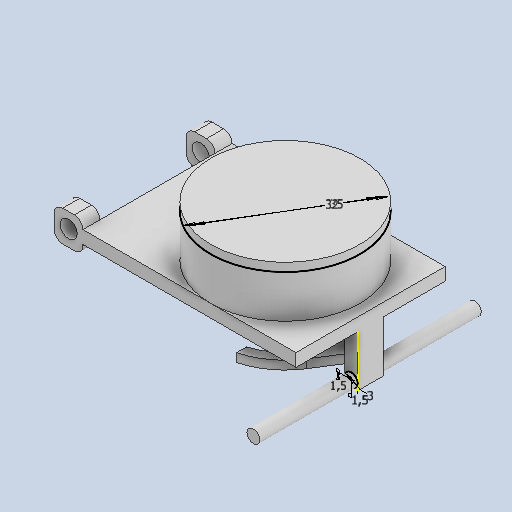
# Autodesk Inventor part: lid
Saved by Autodesk Inventor 2025 (Build 290162000, 162)
## iProperties
Created: 2025-08-06
Part Number: lid
Material: Generic
Document SubType Name: Modeling
Designer: Pravoslav
Density: 1 g/cm^3
Appearance: Default
Author: Pravoslav
Autodesk Inventor part; units mm, degrees
ref_plane "YZ Plane" through (0, 0, 0) normal (1, 0, 0) x (0, 1, 0)
ref_plane "XZ Plane" through (0, 0, 0) normal (0, 1, 0) x (-1, 0, 0)
ref_plane "XY Plane" through (0, 0, 0) normal (0, 0, 1) x (1, 0, 0)
sketch "Sketch1" plane through (0, 0, 0) normal (0, 1, 0) x (-1, 0, 0)
  circle A0 centre (0, 0) radius 16
  circle A1 centre (0, 0) radius 17.5
  dimension "d0" = 32
  dimension "d1" = 35
  constraints: 2 centre point, 2 coincident
  measures "d0" diameter of A0
  measures "d1" diameter of A1
extrude "Extrusion1" add sketch "Sketch1" along normal blind 2 contours A0 | A1
extrude "Extrusion2" add sketch "Sketch1" against normal blind 13
sketch "Sketch2" plane through (0, -13, 0) normal (0, -1, 0) x (1, 0, 0)
  line L0 (20, -17.5) -> (-30, -17.5)
  line L1 (-30, -17.5) -> (-30, 17.5)
  line L2 (-30, 17.5) -> (20, 17.5)
  line L3 (20, 17.5) -> (20, -17.5)
  circle A0 centre (0, 0) radius 17.5 projected
  point P0 (20, 0)
  point P1 (0, 17.5)
  point P2 (0, -17.5)
  point P3 (-9.0139, -15)
  point P4 (-9.0139, 15)
  dimension "d6" = 50
  dimension "d7" = 35
  dimension "d8" = 20
  dimension "d9" = 0
  constraints: 8 end point, 2 parallel, 1 horizontal, 1 midpoint, 1 perpendicular
  measures "d6" distance of L1.end L2.end
  measures "d7" distance of L2.end L0.start
  measures "d8" distance of A0.centre point (20, 0)
  measures "d9" vertical distance of point (0, 0) point (20, 0)
extrude "Extrusion3" add sketch "Sketch2" against normal blind 3 contours L0 A0 L2 L3 | L0 L1 L2 A0
sketch "Sketch3" plane through (-30, -13, 17.5) normal (0, 0, 1) x (1, 0, 0)
  circle A0 centre (-3.3331, 1.4679) radius 2
  line L0 (0, -2.2933) -> (-6.747, -2.2933)
  line L1 (-6.747, -2.2933) -> (-6.747, 4.9975)
  line L2 (-6.747, 4.9975) -> (0, 4.9975)
  line L3 (0, 4.9975) -> (0, -2.2933)
  point P0 (30, 13)
  dimension "d12" = 4
  constraints: 8 end point, 2 parallel, 1 centre point, 1 horizontal, 1 perpendicular
  measures "d12" diameter of A0
extrude "Extrusion4" add sketch "Sketch3" against normal blind 4
fillet "Fillet1" radius 2 4 edges at (-36.747, -8.0025, 15.5) (-30, -8.0025, 15.5) (-36.747, -15.2933, 15.5) (-30, -15.2933, 15.5)
mirror "Mirror1" about plane through (0, 0, 0) normal (0, 0, 1) of "Extrusion4", "Fillet1"
sketch "Sketch5" plane through (0, -13, 0) normal (0, -1, 0) x (1, 0, 0)
  line L0 (20, -17.5) -> (20, 17.5) projected
  line L1 (20, -3) -> (17, -3)
  line L2 (17, -3) -> (17, 3)
  line L3 (17, 3) -> (20, 3)
  line L4 (20, 3) -> (20, -3)
  point P0 (0, 0)
  point P1 (20, 0)
  dimension "d19" = 3
  dimension "d20" = 6
  dimension "d21" = 3
  constraints: 8 end point, 2 parallel, 1 horizontal, 1 midpoint, 1 perpendicular, 1 point on line
  measures "d19" distance from line of L1 point (20, 0)
  measures "d20" distance between parallel lines of L3 L1
  measures "d21" distance between parallel lines of L0 L2
extrude "Extrusion6" add sketch "Sketch5" along normal blind 8
sketch "Sketch6" plane through (0, -21, 0) normal (0, -1, 0) x (1, 0, 0)
  circle A0 centre (0, 0) radius 13.75
  circle A1 centre (0, 0) radius 15.9872
  line L0 (17, -3) -> (17, 3) projected
  line L1 (17, -3) -> (14.1171, -7.5034)
  line L2 (17, 3) -> (13.5326, 8.5123)
  line L3 (4.0303, -16) -> (4.0303, 16.2457)
  point P0 (4.0303, 15.4709)
  point P1 (4.0303, 13.1461)
  point P2 (4.0303, -13.1461)
  point P3 (4.0303, -15.4709)
  dimension "d24" = 27.5
  constraints: 6 end point, 2 centre point, 2 coincident, 2 point on circle, 1 tangent, 1 vertical
  measures "d24" diameter of A0
extrude "Extrusion7" add sketch "Sketch6" against normal blind 2 contours A0 L3 A1 | L2 L0 L1 A1 picked at (5.0608, -14.3101)
sketch "Sketch7" plane through (0, -21, 0) normal (0, -1, 0) x (1, 0, 0)
  line L0 (17, 3) -> (20, 3) projected
  line L1 (17, -3) -> (14.1171, -7.5034) projected
  line L2 (20, 3) -> (17, 3)
  line L3 (17, 3) -> (17, -3)
  line L4 (17, -3) -> (20, -3)
  line L5 (20, -3) -> (20, 3)
  point P0 (0, 0)
  constraints: 8 end point, 2 parallel, 1 horizontal, 1 perpendicular
extrude "Extrusion8" add sketch "Sketch7" along normal blind 4
sketch "Sketch8" plane through (17, -13, 3) normal (0, 0, 1) x (1, 0, 0)
  circle A0 centre (1.5, -10.5) radius 1.5
  line L0 (3, 0) -> (3, -12) projected
  line L1 (3, -12) -> (0, -12) projected
  point P0 (-17, 13)
  dimension "d29" = 3
  dimension "d30" = 1.5
  dimension "d31" = 1.5
  constraints: 1 centre point
  measures "d29" diameter of A0
  measures "d30" distance from line of L0 A0.centre
  measures "d31" distance from line of L1 A0.centre
extrude "Extrusion9" add sketch "Sketch8" along normal blind 23 contours A0
extrude "Extrusion10" add sketch "Sketch8" against normal blind 29 contours A0
body "Solid1"
